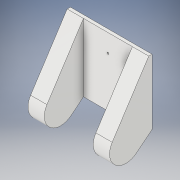
# Autodesk Inventor part: HA004
Saved by Autodesk Inventor 2017 SP1 (Build 210196100, 196)
## iProperties
Created: 2017-06-10
Part Number: HA004
Material: Generic
Document SubType Name: Modeling
Designer: Zach
Density: 1 g/cm^3
Appearance: CR White
Author: Zach
Autodesk Inventor part; units mm, degrees
ref_plane "YZ Plane" through (0, 0, 0) normal (1, 0, 0) x (0, 1, 0)
ref_plane "XZ Plane" through (0, 0, 0) normal (0, 1, 0) x (-1, 0, 0)
sketch "Sketch1" plane through (0, 0, 0) normal (0, 0, 1) x (1, 0, 0)
  line L0 (-125, -100) -> (125, -100)
  line L1 (125, -100) -> (125, 100)
  line L2 (125, 100) -> (-125, 100)
  line L3 (-125, 100) -> (-125, -100)
  line L4 (-125, -100) -> (125, 100) construction
  line L5 (125, -100) -> (-125, 100) construction
  point P0 (0, 0)
  dimension "d0" = 250
  dimension "d1" = 200
  constraints: 12 end point, 2 midpoint, 2 parallel, 1 horizontal, 1 perpendicular
  measures "d0" distance of L2.end L1.end
  measures "d1" distance of L1.end L0.end
extrude "Extrusion1" add sketch "Sketch1" along normal blind 10
sketch "Sketch2" plane through (0, 0, 10) normal (0, 0, 1) x (1, 0, 0)
  circle A0 centre (0, 45) radius 3
  point P0 (0, 0)
  dimension "d13" = 6
  dimension "d14" = 45
  constraints: 1 centre point, 1 vertical alignment
  measures "d13" diameter of A0
  measures "d14" distance of point (0, 0) A0.centre
extrude "Extrusion2" cut sketch "Sketch2" against normal through all
sketch "Sketch4" plane through (125, -100, 0) normal (1, 0, 0) x (0, 0, -1)
  circle A0 centre (-80, 0) radius 50 construction
  line L0 (0, 0) -> (-10, 0)
  line L1 (0, 0) -> (-48.75, -39.0312)
  line L2 (-10, 0) -> (-10, 200)
  line L3 (-10, 200) -> (-121.9627, 27.187)
  arc A1 (-121.9627, 27.187) -> (-48.75, -39.0312) centre (-80, 0) ccw
  line L4 (0, 0) -> (-10, 0)
  line L5 (-10, 200) -> (-10, 0)
  dimension "d8" = 100
  dimension "d20" = 80
  constraints: 12 end point, 4 point on circle, 4 tangent, 3 coincident, 2 centre point, 2 collinear, 1 horizontal alignment
  measures "d8" diameter of A0
  measures "d20" distance of point (0, 0) A0.centre
extrude "Extrusion3" add sketch "Sketch4" against normal blind 250
ref_plane "Work Plane1" through (0, 0, 10) normal (0, 0, 1) x (1, 0, 0)
sketch "Sketch5" plane through (0, 0, 10) normal (0, 0, 1) x (1, 0, 0)
  line L0 (125, 100) -> (-125, 100) projected
  line L1 (125, -150) -> (-125, -150) projected
  line L2 (-75, 100) -> (75, 100)
  line L3 (75, 100) -> (75, -150)
  line L4 (75, -150) -> (-75, -150)
  line L5 (-75, -150) -> (-75, 100)
  line L6 (-125, 100) -> (-125, -100) projected
  line L7 (125, -100) -> (125, 100) projected
  point P0 (0, 0)
  dimension "d16" = 50
  dimension "d17" = 50
  constraints: 8 end point, 2 parallel, 2 point on line, 1 horizontal, 1 perpendicular
  measures "d16" distance between parallel lines of L6 L5
  measures "d17" distance between parallel lines of L7 L3
extrude "Extrusion4" cut sketch "Sketch5" along normal through all
body "Solid1"
